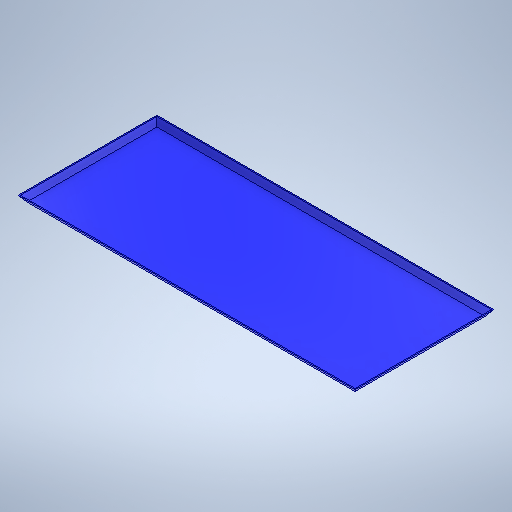
# Autodesk Inventor part: ChipTray
Saved by Autodesk Inventor 2025 (Build 290162010, 162A)
## iProperties
Created: 2024-08-20
Part Number: ChipTray
Material: Generic
Document SubType Name: Modeling
Designer: max_d
Density: 1 g/cm^3
Appearance: Default
Author: max_d
Autodesk Inventor part; units mm, degrees
ref_plane "YZ Plane" through (0, 0, 0) normal (1, 0, 0) x (0, 1, 0)
ref_plane "XY Plane" through (0, 0, 0) normal (0, 0, 1) x (1, 0, 0)
sketch "Sketch1" plane through (0, 0, 0) normal (0, 1, 0) x (-1, 0, 0)
  line L0 (552.5, 227.5) -> (-552.5, 227.5)
  line L1 (-552.5, 227.5) -> (-552.5, -227.5)
  line L2 (-552.5, -227.5) -> (552.5, -227.5)
  line L3 (552.5, -227.5) -> (552.5, 227.5)
  line L4 (552.5, 227.5) -> (-552.5, -227.5) construction
  line L5 (-552.5, 227.5) -> (552.5, -227.5) construction
  point P0 (0, 0)
  dimension "d0" = 1105
  dimension "d1" = 455
  constraints: 12 end point, 2 midpoint, 2 parallel, 1 horizontal, 1 perpendicular
  measures "d0" distance of L2.end L1.end
  measures "d1" distance of L1.end L0.end
ref_plane "Work Plane1" through (0, -20, 0) normal (0, 1, 0) x (-1, 0, 0)
sketch "Sketch2" plane through (0, -20, 0) normal (0, 1, 0) x (-1, 0, 0)
  line L0 (-537.5, 212.5) -> (537.5, 212.5)
  line L1 (537.5, 212.5) -> (537.5, -212.5)
  line L2 (537.5, -212.5) -> (-537.5, -212.5)
  line L3 (-537.5, -212.5) -> (-537.5, 212.5)
  line L4 (-537.5, 212.5) -> (537.5, -212.5) construction
  line L5 (537.5, 212.5) -> (-537.5, -212.5) construction
  point P0 (0, 0)
  dimension "d3" = 1075
  dimension "d4" = 425
  constraints: 12 end point, 2 midpoint, 2 parallel, 1 horizontal, 1 perpendicular
  measures "d3" distance of L1.end L2.end
  measures "d4" distance of L0.end L1.end
loft "Loft1" add profiles "Sketch1", "Sketch2"
shell "Shell1" thickness 3 removed faces 1 at (184.1667, 0, 75.8333)
body "Solid1"
